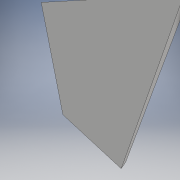
# Autodesk Inventor part: Simulation
Saved by Autodesk Inventor 2018 (Build 220112000, 112)
## iProperties
Created: 2018-09-02
Part Number: Simulation
Material: Generic
Document SubType Name: Modeling
Designer: matth
Density: 1 g/cm^3
Appearance: Default
Author: matth
Autodesk Inventor part; units mm, degrees
ref_plane "YZ Plane" through (0, 0, 0) normal (1, 0, 0) x (0, 1, 0)
ref_plane "XZ Plane" through (0, 0, 0) normal (0, 1, 0) x (-1, 0, 0)
ref_plane "XY Plane" through (0, 0, 0) normal (0, 0, 1) x (1, 0, 0)
sketch "Sketch1" plane through (0, 0, 0) normal (0, 1, 0) x (-1, 0, 0)
  line L0 (0, 0) -> (1820, 0)
  line L1 (1820, 0) -> (1820, -2430)
  line L2 (1820, -2430) -> (0, -2430)
  line L3 (0, -2430) -> (0, 0)
  dimension "d0" = 1820
  dimension "d1" = 2430
  constraints: 8 end point, 2 parallel, 1 horizontal, 1 perpendicular
  measures "d0" distance of L1.end L2.end
  measures "d1" distance of L0.end L1.end
extrude "Extrusion1" add sketch "Sketch1" along normal blind 50
sketch "Sketch2" plane through (0, 50, 0) normal (0, 1, 0) x (1, 0, 0)
  line L0 (-1820, 2430) -> (-1820, 0) projected
  line L1 (-1820, 0) -> (-1820, 250)
  line L2 (-1820, 250) -> (-1570, 250)
  line L3 (-1820, 250) -> (-1570, 250) construction
  line L4 (0, 2430) -> (-1820, 2430) projected
  line L5 (0, 2430) -> (0, 2180)
  line L6 (0, 0) -> (0, 2430) projected
  line L7 (0, 2180) -> (-250, 2180)
  line L8 (-1570, 250) -> (-250, 250)
  line L9 (-250, 250) -> (-250, 2180)
  line L10 (-250, 2180) -> (-1570, 2180)
  line L11 (-1570, 2180) -> (-1570, 250)
  line L12 (-1570, 250) -> (-1570, 300)
  line L13 (-1570, 300) -> (-1520, 300)
  line L14 (-250, 2180) -> (-300, 2180)
  line L15 (-300, 2180) -> (-300, 2130)
  line L16 (-1520, 300) -> (-300, 300)
  line L17 (-300, 300) -> (-300, 2130)
  line L18 (-300, 2130) -> (-1520, 2130)
  line L19 (-1520, 2130) -> (-1520, 300)
  dimension "d4" = 250
  dimension "d5" = 250
  dimension "d6" = 0
  dimension "d7" = 250
  dimension "d8" = 250
  dimension "d9" = 50
  dimension "d10" = 50
  dimension "d11" = 50
  dimension "d12" = 50
  constraints: 34 end point, 5 perpendicular, 4 horizontal, 4 parallel, 4 point on line, 1 collinear
  measures "d4" distance of L0.end L1.end
  measures "d5" distance of L1.end L2.end
  measures "d6" distance between parallel lines of L2 L3
  measures "d7" distance of L4.start L5.end
  measures "d8" distance of L5.end L7.end
  measures "d9" distance of L3.end L12.end
  measures "d10" distance of L12.end L13.end
  measures "d11" distance of L7.end L14.end
  measures "d12" distance of L14.end L15.end
extrude "Extrusion2" cut sketch "Sketch2" against normal blind 0.001 contours L11 L13 L16 L17 L15 L10 L9 L8 | L11 L10 L15 L18 L19 L13
sketch "Sketch3" plane through (0, 0, 0) normal (0, -1, 0) x (1, 0, 0)
  line L0 (0, -2430) -> (-1820, -2430) projected
  line L1 (0, 0) -> (-1820, 0)
  line L2 (-1820, 0) -> (-1820, -2430)
  line L3 (-1820, -2430) -> (0, -2430)
  line L4 (0, -2430) -> (0, 0)
  line L5 (0, 0) -> (20, 0)
  line L6 (20, 0) -> (20, 20)
  line L7 (20, 20) -> (-1840, 20)
  line L8 (-1840, 20) -> (-1840, -2450)
  line L9 (-1840, -2450) -> (20, -2450)
  line L10 (20, -2450) -> (20, 20)
  dimension "d15" = 20
  dimension "d16" = 20
  dimension "d17" = 1860
  dimension "d18" = 2470
  constraints: 20 end point, 4 parallel, 3 horizontal, 3 perpendicular
  measures "d15" distance of L1.start L5.end
  measures "d16" distance of L5.end L6.end
  measures "d17" distance of L9.end L8.end
  measures "d18" distance of L8.end L7.end
extrude "Extrusion3" add sketch "Sketch3" against normal blind 150
sketch "Sketch4" plane through (0, 50, 0) normal (0, 1, 0) x (1, 0, 0)
  line L0 (-300, 300) -> (-300, 2130) projected
  line L1 (-300, 1215) -> (-910, 1215)
  line L2 (-300, 2130) -> (-1520, 2130) projected
  line L3 (-910, 1215) -> (-910, 2130)
  line L4 (-1570, 2180) -> (-250, 2180) projected
  line L5 (-910, 2130) -> (-1135, 2130)
  line L6 (-1135, 2130) -> (-1135, 2204)
  line L7 (-1135, 2130) -> (-1145, 2130)
  line L8 (-1145, 2130) -> (-1145, 2214)
  line L9 (-1145, 2214) -> (-1135, 2214)
  line L10 (-1135, 2214) -> (-1135, 2130)
  line L11 (-1135, 2214) -> (-675, 2214)
  line L12 (-675, 2214) -> (-675, 2204)
  line L13 (-675, 2204) -> (-1135, 2204)
  line L14 (-1135, 2204) -> (-1135, 2214)
  line L15 (-675, 2204) -> (-685, 2204)
  line L16 (-685, 2204) -> (-685, 2130)
  line L17 (-685, 2130) -> (-675, 2130)
  line L18 (-675, 2130) -> (-675, 2204)
  line L19 (-300, 300) -> (-1520, 300)
  line L20 (-1135, 300) -> (-1135, 226)
  line L21 (-1135, 300) -> (-1145, 300)
  line L22 (-1145, 300) -> (-1145, 216)
  line L23 (-1145, 216) -> (-1135, 216)
  line L24 (-1135, 216) -> (-675, 216)
  line L25 (-675, 216) -> (-675, 226)
  line L26 (-675, 226) -> (-1135, 226)
  line L27 (-685, 226) -> (-685, 300)
  line L28 (-685, 300) -> (-675, 300)
  line L29 (-675, 300) -> (-675, 226)
  line L30 (-1145, 216) -> (-675, 216)
  line L31 (-675, 216) -> (-675, 226)
  line L32 (-675, 226) -> (-1145, 226)
  line L33 (-1145, 226) -> (-1145, 216)
  line L34 (-675, 226) -> (-685, 226)
  line L35 (-685, 226) -> (-685, 300)
  line L36 (-685, 300) -> (-675, 300)
  line L37 (-675, 300) -> (-675, 226)
  line L38 (-1145, 226) -> (-1135, 226)
  line L39 (-1135, 226) -> (-1135, 300)
  line L40 (-1135, 300) -> (-1145, 300)
  line L41 (-1145, 300) -> (-1145, 226)
  point P0 (0, 0)
  dimension "d22" = 225
  dimension "d23" = 74
  dimension "d24" = 10
  dimension "d25" = 84
  dimension "d26" = 460
  dimension "d27" = 10
  constraints: 78 end point, 13 parallel, 12 symmetric about line, 7 perpendicular, 6 horizontal, 4 point on line, 2 midpoint
  measures "d22" distance of L3.end L5.end
  measures "d23" distance of L5.end L6.end
  measures "d24" distance of L8.end L9.end
  measures "d25" distance of L7.end L8.end
  measures "d26" distance of L12.end L13.end
  measures "d27" distance of L17.end L16.end
extrude "Extrusion4" add sketch "Sketch4" along normal blind 140 contours L2 L16 L4 L18 | L4 L16 L13 L18 | L2 L8 L4 L6 | L13 L10 L11 L12 | L4 L8 L9 L10 L6 | L29 L26 L27 L19 | L25 L24 L23 L22 L32 L26 | L20 L32 L22 L19
sketch "Sketch5" plane through (0, 190, 0) normal (0, 1, 0) x (1, 0, 0)
  line L0 (-1145, 300) -> (-1145, 250) projected
  line L1 (-675, 250) -> (-675, 300) projected
  line L2 (-1145, 300) -> (-675, 300)
  line L3 (-675, 300) -> (-675, 280)
  line L4 (-675, 280) -> (-1145, 280)
  line L5 (-1145, 280) -> (-1145, 300)
  line L6 (-300, 2130) -> (-1520, 2130) projected
  line L7 (-675, 2130) -> (-675, 2180) projected
  line L8 (-1145, 2130) -> (-675, 2130)
  line L9 (-675, 2130) -> (-675, 2150)
  line L10 (-675, 2150) -> (-1145, 2150)
  line L11 (-1145, 2150) -> (-1145, 2130)
  line L12 (-1145, 2180) -> (-1145, 2130) projected
  line L13 (-1145, 2130) -> (-675, 2130)
  line L14 (-675, 2130) -> (-675, 2130.001)
  line L15 (-675, 2130.001) -> (-1145, 2130.001)
  line L16 (-1145, 2130.001) -> (-1145, 2130)
  line L17 (-1135, 300) -> (-1145, 300) projected
  line L18 (-675, 216) -> (-675, 300) projected
  line L19 (-1145, 300) -> (-675, 300)
  line L20 (-675, 300) -> (-675, 299.999)
  line L21 (-675, 299.999) -> (-1145, 299.999)
  line L22 (-1145, 299.999) -> (-1145, 300)
  point P0 (0, 0)
  dimension "d30" = 20
  dimension "d31" = 20
  dimension "d34" = 0.001
  dimension "d35" = 0.001
  constraints: 32 end point, 8 parallel, 6 point on line, 4 horizontal, 4 perpendicular
  measures "d30" distance of L2.end L3.end
  measures "d31" distance of L9.end L8.end
  measures "d34" distance of L14.end L13.end
  measures "d35" distance of L19.end L20.end
extrude "Extrusion5" add sketch "Sketch5" along normal blind 20
sketch "Sketch6" plane through (0, 50, 0) normal (0, 1, 0) x (1, 0, 0)
  line L0 (-1520, 300) -> (-1145, 300) projected
  circle A0 centre (-1520, 300) radius 105
  line L1 (-1135, 300) -> (-685, 300) projected
  line L2 (-910, 300) -> (-910, 415)
  circle A1 centre (-910, 415) radius 105
  line L3 (-300, 300) -> (-300, 2130) projected
  circle A2 centre (-300, 300) radius 105
  point P0 (0, 0)
  dimension "d36" = 210
  dimension "d37" = 115
  dimension "d38" = 210
  dimension "d39" = 210
  constraints: 3 centre point, 2 end point, 1 coincident, 1 midpoint, 1 vertical
  measures "d36" diameter of A0
  measures "d37" distance of L2.start L2.end
  measures "d38" diameter of A1
  measures "d39" diameter of A2
extrude "Extrusion6" add sketch "Sketch6" along normal blind 115
sketch "Sketch7" plane through (-1520, 165, -300) normal (0, 1, 0) x (1, 0, 0)
  circle A0 centre (610, 115) radius 105 projected
  line L0 (610, 115) -> (590, 115)
  line L1 (590, 115) -> (590, 136.6505)
  line L2 (590, 136.6505) -> (630, 136.6505)
  line L3 (630, 136.6505) -> (630, 93.3495)
  line L4 (630, 93.3495) -> (590, 93.3495)
  line L5 (590, 93.3495) -> (590, 115)
  point P0 (1520, -300)
  dimension "d42" = 20
  dimension "d43" = 21.6505
  dimension "d44" = 40
  dimension "d45" = 43.301
  constraints: 12 end point, 5 perpendicular, 1 horizontal, 1 point on line
  measures "d42" distance of L0.start L0.end
  measures "d43" distance of L0.end L1.end
  measures "d44" distance of L1.end L2.end
  measures "d45" distance of L2.end L3.end
extrude "Extrusion7" add sketch "Sketch7" along normal blind 81.5 contours L1 L2 L3 L4 L5
sketch "Sketch8" plane through (-890, 165, -393.3495) normal (1, 0, 0) x (0, 0, -1)
  line L0 (43.301, 81.5) -> (0, 81.5) projected
  line L1 (21.6505, 81.5) -> (21.6505, 69)
  line L2 (21.6505, 69) -> (43.301, 81.5)
  line L3 (21.6505, 69) -> (0, 81.5)
  line L4 (0, 81.5) -> (0, 0)
  line L5 (126.6505, 0) -> (-83.3495, 0) projected
  line L6 (43.301, 0) -> (43.301, 81.5) projected
  line L7 (0, 0) -> (43.301, 0)
  line L8 (43.301, 0) -> (43.301, 81.5)
  point P0 (-393.3495, -165)
  dimension "d48" = 12.5
  constraints: 12 end point, 2 vertical, 1 collinear, 1 horizontal, 1 midpoint, 1 point on line
  measures "d48" distance of L1.start L1.end
extrude "Extrusion8" cut sketch "Sketch8" against normal blind 40 contours L6 L5 L4 L3 L2
sketch "Sketch9" plane through (-910, 165, -415) normal (0, 1, 0) x (1, 0, 0)
  circle A0 centre (0, 0) radius 2.5
  point P0 (910, -415)
  dimension "d51" = 5
  constraints: 1 centre point
  measures "d51" diameter of A0
extrude "Extrusion9" add sketch "Sketch9" along normal blind 49
sketch "Sketch10" plane through (-910, 214, -415) normal (0, 1, 0) x (1, 0, 0)
  line L0 (20, 0) -> (-20, 0) projected
  line L1 (0, 0) -> (2.9883, 0)
  line L2 (2.9883, 0) -> (2.9883, -4.9362)
  line L3 (2.9883, -4.9362) -> (0, -4.9362)
  line L4 (0, -4.9362) -> (0, 0)
  line L5 (0, 0) -> (4.3041, 0)
  line L6 (4.3041, 0) -> (4.3041, 5.8291)
  line L7 (4.3041, 5.8291) -> (0, 5.8291)
  line L8 (0, 5.8291) -> (0, 0)
  point P0 (910, -415)
  constraints: 16 end point, 4 parallel, 2 horizontal, 2 perpendicular, 1 midpoint
extrude "Extrusion10" cut sketch "Sketch10" against normal blind 49
sketch "Sketch11" plane through (-910, 214, -412.5) normal (1, 0, 0) x (0, 0, -1)
  line L0 (5, 0) -> (0, 0) projected
  line L1 (2.5, 0) -> (2.5, -5)
  line L2 (2.5, -5) -> (5, -5)
  line L3 (5, 0) -> (5, -49) projected
  line L4 (2.5, 0) -> (5, -5)
  line L5 (2.5, -5) -> (0, -5)
  line L6 (0, -49) -> (0, 0) projected
  line L7 (0, -5) -> (2.5, 0)
  line L8 (2.5, 0) -> (0, 0)
  line L9 (0, 0) -> (0, -5)
  line L10 (2.5, 0) -> (5, 0)
  line L11 (5, 0) -> (5, -5)
  point P0 (-412.5, -214)
  dimension "d56" = 5
  constraints: 18 end point, 4 point on line, 3 perpendicular, 1 horizontal, 1 midpoint, 1 vertical
  measures "d56" distance of L1.start L1.end
extrude "Extrusion11" cut sketch "Sketch11" against normal blind 49 contours L3 L4 L0 | L7 L6 L0
sketch "Sketch12" plane through (-910, 165, -412.5) normal (1, 0, 0) x (0, 0, -1)
  line L0 (0, 0) -> (0, 44) projected
  line L1 (5, 44) -> (2.5, 49) projected
  line L2 (0, 44) -> (2.5, 49)
  line L3 (2.5, 49) -> (0, 49)
  line L4 (0, 49) -> (0, 44)
  line L5 (2.5, 49) -> (2.5, 44)
  point P0 (-412.5, -165)
  constraints: 8 end point, 1 horizontal, 1 perpendicular, 1 vertical
revolve "Revolution1" cut sketch "Sketch12" angle 360 about axis through (-910, 214, -415) along (0, -1, 0)
sketch "Sketch13" plane through (-910, 165, -412.5) normal (1, 0, 0) x (0, 0, -1)
  line L0 (2.5, 49) -> (0, 44) projected
  line L1 (2.5, 49) -> (2.5, 0)
  line L2 (0, 0) -> (5, 0) projected
  line L3 (0, 0) -> (2.5, 0)
  line L4 (0, 0) -> (0, 44) projected
  line L5 (0, 0) -> (0, 44)
  line L6 (0, 44) -> (2.5, 49)
  point P0 (-412.5, -165)
  constraints: 8 end point, 1 midpoint, 1 perpendicular, 1 vertical
revolve "Revolution2" add sketch "Sketch13" angle 360 about axis through (-910, 214, -415) along (0, -1, 0)
body "Solid1"
